fhl_award (Autodesk Fusion 360 design; units mm, degrees)
Autodesk Fusion 360 part; units mm, degrees
note: some values were not read from the file. Set by a fixed rule: which sketch regions a step uses.
(part 1 of 2)
sketch "Sketch1" plane through (0, 0, 0) normal (0, 1, 0) x (1, 0, 0)
  line L0 (0, 0) -> (-70, 0)
  line L1 (-70, 0) -> (-70, -200)
  line L2 (-70, -200) -> (0, -200)
  line L3 (0, -200) -> (0, 0)
  line L4 (-63, -200) -> (-7, -200)
  line L5 (-63, -200) -> (-11.8843, -162.1937)
  line L6 (-11.8843, -162.1937) -> (-35, -218)
  line L7 (-35, -218) -> (-66.1664, -152.3416)
  line L8 (-66.1664, -152.3416) -> (-7, -200)
  line L9 (-35, -218) -> (-35, -200)
  line L10 (-43.5442, -200) -> (-27.5442, -200)
  dimension "d1" = 70
  dimension "d2" = 200
  dimension "d3" = 7
  dimension "d4" = 7
  dimension "d5" = 18
  dimension "d6" = 16
  dimension "d7" = 112.5
  dimension "d9" = 101.095
  dimension "d10" = 106.351
  constraint horizontal L0
  constraint vertical L1
  constraint horizontal L2
  constraint vertical L3
  constraint coincident L0.start L3.end
  constraint coincident L2 L4.start
  constraint coincident L2 L4.end
  constraint perpendicular L2 L9
  constraint midpoint L2 L9.end
  constraint coincident L7 L10.start
  constraint coincident L6 L10.end
  constraint collinear L4 L10
  measures "d1" distance of L1.end L2.end
  measures "d2" distance of L0.start L2.end
  measures "d3" distance of L2.end L4.end
  measures "d4" distance of L1.end L4.start
  measures "d5" distance of L2 L6.end
  measures "d6" distance of L10.start L10.end
  measures "d7" angle of L2 L6
  measures "d9" angle of L5 L7
  measures "d10" angle of L6 L8
extrude "Extrude1" add sketch "Sketch1" along normal blind 48 contours L0 L1 L2 L3 L5 L6 L7 L8 | L2 L4 L6 L8 | L2 L4 L5 L7 | L2 L4 L5 L6 L7 L8 L10 | L5 L6 L8 | L5 L7 L8
extrude "Extrude2" add sketch "Sketch1" against normal blind 8 contours L2 L4 L6 L8 | L2 L4 L5 L7 | L2 L4 L6 L9 L10 | L2 L4 L5 L6 L7 L8 L10 | L5 L6 L8 | L2 L4 L7 L9 L10 | L5 L7 L8
sketch "Sketch2" plane through (-70, 0, 0) normal (-1, 0, 0) x (0, -1, 0)
  line L0 (0, 0) -> (0, 200)
  line L1 (0, 200) -> (-48, 200)
  line L2 (-48, 200) -> (-48, 0)
  line L3 (-48, 0) -> (0, 0)
  line L4 (-4, 200) -> (-48, 11.1856)
  line L5 (0, 0) -> (-48, 11.1856)
  line L6 (-4, 200) -> (-48, 200)
  line L7 (-48, 200) -> (-48, 0)
  line L8 (-48, 0) -> (0, 0)
  point P0 (0, 200)
  dimension "d15" = 90
  dimension "d16" = 4
  constraint coincident L1 L4.start
  constraint coincident L2 L4.end
  constraint coincident L0.start L3.end
  constraint coincident L1.end L2.start
  constraint coincident L2.end L3.start
  measures "d15" angle of L4 L5
  measures "d16" distance of L4.start P0
extrude "Extrude3" cut sketch "Sketch2" against normal blind 70 contours L2 L3 L5 L7 L8 | L1 L2 L4 L6 L7
fillet "Fillet1" radius 1 29 edges at (-70, 0, 100) (0, 26, 105.5928) (-35, 48, 11.1856) (-70, 26, 105.5928) (-70, 24, 5.5928) (-35, 4, 200) (-70, 2, 200) (0, 0, 100) (-3.5, 0, 200) (-7, -4, 200) (-63, -4, 200) (-66.5, 0, 200) (-55.7999, -8, 194.6746) (-53.2721, -8, 200) (-39.2721, -8, 209) (-35, -4, 218) (-39.2721, 0, 209) (-31.2721, 0, 209) (-31.2721, -8, 209) (-17.2721, -8, 200) (-14.7022, -8, 193.7959) (-57.3831, -8, 170.8455) (-49.9863, -8, 165.3746) (-22.8453, -8, 170.3007) (-17.1444, -8, 174.8927) (-66.1664, -4, 152.3416) (-11.8843, -4, 162.1937) (-35, 0, 0) (0, 24, 5.5928)
sketch "Sketch3" plane through (0, 0, 0) normal (0, -1, 0) x (1, 0, 0)
  line L0 (-1, 199) -> (-8.8356, 199)
  arc A0 (-9.2083, 198.2212) -> (-8.8356, 199) centre (-9.8356, 199) ccw
  line L1 (-9.2083, 198.2212) -> (-22.4045, 187.5917)
  line L2 (-22.4045, 187.5917) -> (-13.2636, 165.5237)
  arc A1 (-14.7821, 164.337) -> (-13.2636, 165.5237) centre (-14.1875, 165.141) ccw
  line L3 (-14.7821, 164.337) -> (-33.8062, 178.4077)
  line L4 (-33.8062, 178.4077) -> (-62.7601, 155.0854)
  arc A2 (-64.2908, 156.293) -> (-62.7601, 155.0854) centre (-63.3874, 155.8642) ccw
  line L5 (-64.2908, 156.293) -> (-48.5998, 189.3493)
  line L6 (-48.5998, 189.3493) -> (-60.5609, 198.196)
  arc A3 (-60.9663, 199) -> (-60.5609, 198.196) centre (-59.9663, 199) ccw
  line L7 (-60.9663, 199) -> (-69, 199)
  line L8 (-69, 199) -> (-69, 1.2598)
  line L9 (-69, 1.2598) -> (-1, 1.2598)
  line L10 (-1, 1.2598) -> (-1, 199)
  line L11 (-62.5, 91.2598) -> (-7.5, 91.2598)
  line L12 (-7.5, 91.2598) -> (-7.5, 71.2598)
  line L13 (-7.5, 71.2598) -> (-62.5, 71.2598)
  line L14 (-62.5, 71.2598) -> (-62.5, 91.2598)
  line L15 (-37.5, 101.2598) -> (-32.5, 101.2598)
  line L16 (-32.5, 101.2598) -> (-32.5, 61.2598)
  line L17 (-32.5, 61.2598) -> (-37.5, 61.2598)
  line L18 (-37.5, 61.2598) -> (-37.5, 101.2598)
  line L19 (-32.5, 61.2598) -> (-7.5, 71.2598)
  line L20 (-7.5, 91.2598) -> (-32.5, 101.2598)
  line L21 (-37.5, 101.2598) -> (-62.5, 91.2598)
  line L22 (-62.5, 71.2598) -> (-37.5, 61.2598)
  line L23 (-35, 101.2598) -> (-35, 61.2598)
  line L24 (-35, 61.2598) -> (-37.5, 61.2598)
  line L25 (-36.25, 61.2598) -> (-36.25, 71.2598)
  line L26 (-35, 61.2598) -> (-32.5, 61.2598)
  line L27 (-33.75, 61.2598) -> (-33.75, 71.2598)
  circle A4 centre (-35, 68.2598) radius 3
  line L28 (-35, 68.2598) -> (-36.25, 68.2598)
  line L29 (-35, 68.2598) -> (-33.75, 68.2598)
  line L30 (-50.0254, 86.3798) -> (-50.0254, 82.5627)
  line L31 (-50.0254, 82.5627) -> (-44.7683, 82.5627)
  line L32 (-44.7683, 82.5627) -> (-44.7683, 79.7284)
  line L33 (-44.7683, 79.7284) -> (-50.0254, 79.7284)
  line L34 (-50.0254, 79.7284) -> (-50.0254, 73.2598)
  line L35 (-50.0254, 73.2598) -> (-54.0254, 73.2598)
  line L36 (-54.0254, 73.2598) -> (-54.0254, 89.2598)
  line L37 (-54.0254, 89.2598) -> (-43.8083, 89.2598)
  line L38 (-43.8083, 89.2598) -> (-43.8083, 86.3798)
  line L39 (-43.8083, 86.3798) -> (-50.0254, 86.3798)
  line L40 (-28.5397, 73.2598) -> (-32.5397, 73.2598)
  line L41 (-32.5397, 73.2598) -> (-32.5397, 79.8884)
  line L42 (-32.5397, 79.8884) -> (-37.454, 79.8884)
  line L43 (-37.454, 79.8884) -> (-37.454, 73.2598)
  line L44 (-37.454, 73.2598) -> (-41.454, 73.2598)
  line L45 (-41.454, 73.2598) -> (-41.454, 89.2598)
  line L46 (-41.454, 89.2598) -> (-37.454, 89.2598)
  line L47 (-37.454, 89.2598) -> (-37.454, 82.9741)
  line L48 (-37.454, 82.9741) -> (-32.5397, 82.9741)
  line L49 (-32.5397, 82.9741) -> (-32.5397, 89.2598)
  line L50 (-32.5397, 89.2598) -> (-28.5397, 89.2598)
  line L51 (-28.5397, 89.2598) -> (-28.5397, 73.2598)
  line L52 (-14.5969, 76.2998) -> (-14.5969, 73.2598)
  line L53 (-14.5969, 73.2598) -> (-24.6083, 73.2598)
  line L54 (-24.6083, 73.2598) -> (-24.6083, 89.2598)
  line L55 (-24.6083, 89.2598) -> (-20.6083, 89.2598)
  line L56 (-20.6083, 89.2598) -> (-20.6083, 76.2998)
  line L57 (-20.6083, 76.2998) -> (-14.5969, 76.2998)
  dimension "d22" = 5
  dimension "d24" = 55
  dimension "d25" = 6.5
  dimension "d26" = 27.5
  dimension "d27" = 40
  dimension "d28" = 70
  dimension "d29" = 20
  dimension "d30" = 10
  dimension "d31" = 3
  constraint horizontal L11
  constraint vertical L12
  constraint horizontal L13
  constraint vertical L14
  constraint horizontal L15
  constraint vertical L16
  constraint horizontal L17
  constraint vertical L18
  constraint midpoint L15 L23.start
  constraint midpoint L17 L23.end
  constraint midpoint L24 L25.start
  constraint coincident L13 L25.end
  constraint perpendicular L13 L25
  constraint midpoint L26 L27.start
  constraint coincident L13 L27.end
  constraint perpendicular L13 L27
  constraint coincident L23 A4.centre
  constraint tangent L13 A4
  constraint coincident A4.centre L28.start
  constraint coincident L25 L28.end
  constraint perpendicular L25 L28
  constraint coincident L27 L29.end
  constraint perpendicular L27 L29
  measures "d22" distance of L16 L18
  measures "d24" distance of L12 L14
  measures "d25" distance of L10 L12
  measures "d26" distance of L12 L23
  measures "d27" distance of L23.start L23.end
  measures "d28" distance of L9 L13
  measures "d29" distance of L11.end L12.end
  measures "d30" distance of L13 L17
  measures "d31" distance of L13 A4.centre
extrude "Extrude4" cut sketch "Sketch3" against normal blind 2 contours L11 L18 L21 | L11 L13 L14 L18 L44 L45 L46 | L11 L15 L18 L23 | L11 L18 L23 L46 L47 L48 | L13 L18 L22 A4 | L11 L15 L16 L23 | L11 L16 L23 L48 L49 L50 | L13 L18 L23 L42 L43 L44 | L13 L18 L25 A4 | L17 L18 L24 L25 A4 | L11 L16 L20 | L11 L12 L13 L16 L40 L50 L51 | L13 L25 A4 | L13 L16 L23 L40 L41 L42 | L23 L27 A4 L29 | L13 L27 A4 | L23 L25 A4 L28 | L13 L16 L19 A4 | L13 L16 L27 A4 | L16 L17 L26 L27 A4 picked at (-34.1667, 69.1689) picked at (-35.8333, 69.1689)
fillet "Fillet3" radius 4 8 edges at (-62.5, 1, 71.2598) (-62.5, 1, 91.2598) (-37.5, 1, 101.2598) (-32.5, 1, 101.2598) (-7.5, 1, 91.2598) (-7.5, 1, 71.2598) (-32.5, 1, 61.2598) (-37.5, 1, 61.2598)
fillet "Fillet4" radius 0.7 4 edges at (-36.25, 1, 68.2598) (-33.75, 1, 68.2598) (-36.25, 1, 65.5326) (-33.75, 1, 65.5326)
fillet "Fillet5" radius 0.7 2 edges at (-33.75, 1, 61.2598) (-36.25, 1, 61.2598)
fillet "Fillet6" radius 0.1 2 edges at (-36.25, 1, 70.987) (-33.75, 1, 70.987)
fillet "Fillet7" radius 0.25 28 edges at (-28.5397, 1, 73.2598) (-32.5397, 1, 73.2598) (-37.454, 1, 73.2598) (-37.454, 1, 79.8884) (-32.5397, 1, 79.8884) (-41.454, 1, 73.2598) (-41.454, 1, 89.2598) (-37.454, 1, 89.2598) (-37.454, 1, 82.9741) (-32.5397, 1, 82.9741) (-32.5397, 1, 89.2598) (-28.5397, 1, 89.2598) (-24.6083, 1, 89.2598) (-20.6083, 1, 89.2598) (-20.6083, 1, 76.2998) (-14.5969, 1, 76.2998) (-14.5969, 1, 73.2598) (-24.6083, 1, 73.2598) (-54.0254, 1, 73.2598) (-54.0254, 1, 89.2598) (-43.8083, 1, 89.2598) (-43.8083, 1, 86.3798) (-50.0254, 1, 82.5627) (-44.7683, 1, 82.5627) (-50.0254, 1, 86.3798) (-44.7683, 1, 79.7284) (-50.0254, 1, 79.7284) (-50.0254, 1, 73.2598)
sketch "Sketch4" plane through (0, 0, 0) normal (0, -1, 0) x (1, 0, 0)
  line L0 (-1, 199) -> (-8.8356, 199)
  arc A0 (-9.2083, 198.2212) -> (-8.8356, 199) centre (-9.8356, 199) ccw
  line L1 (-9.2083, 198.2212) -> (-22.4045, 187.5917)
  line L2 (-22.4045, 187.5917) -> (-13.2636, 165.5237)
  arc A1 (-14.7821, 164.337) -> (-13.2636, 165.5237) centre (-14.1875, 165.141) ccw
  line L3 (-14.7821, 164.337) -> (-33.8062, 178.4077)
  line L4 (-33.8062, 178.4077) -> (-62.7601, 155.0854)
  arc A2 (-64.2908, 156.293) -> (-62.7601, 155.0854) centre (-63.3874, 155.8642) ccw
  line L5 (-64.2908, 156.293) -> (-48.5998, 189.3493)
  line L6 (-48.5998, 189.3493) -> (-60.5609, 198.196)
  arc A3 (-60.9663, 199) -> (-60.5609, 198.196) centre (-59.9663, 199) ccw
  line L7 (-60.9663, 199) -> (-69, 199)
  line L8 (-69, 199) -> (-69, 1.2598)
  line L9 (-69, 1.2598) -> (-1, 1.2598)
  line L10 (-1, 1.2598) -> (-1, 199)
  arc A4 (-33.6034, 70.9149) -> (-33.75, 70.8264) centre (-33.65, 70.8264) ccw
  line L11 (-33.75, 70.8264) -> (-33.75, 68.9598)
  arc A5 (-34.45, 68.2598) -> (-33.75, 68.9598) centre (-34.45, 68.9598) ccw
  line L12 (-34.45, 68.2598) -> (-35.55, 68.2598)
  arc A6 (-36.25, 68.9598) -> (-35.55, 68.2598) centre (-35.55, 68.9598) ccw
  line L13 (-36.25, 68.9598) -> (-36.25, 70.8264)
  arc A7 (-36.25, 70.8264) -> (-36.3966, 70.9149) centre (-36.35, 70.8264) ccw
  arc A8 (-36.3966, 70.9149) -> (-36.5811, 65.7103) centre (-35, 68.2598) ccw
  arc A9 (-36.25, 65.1154) -> (-36.5811, 65.7103) centre (-36.95, 65.1154) ccw
  line L14 (-36.25, 65.1154) -> (-36.25, 61.9672)
  arc A10 (-36.9967, 61.2688) -> (-36.25, 61.9672) centre (-36.95, 61.9672) ccw
  arc A11 (-38.2152, 61.5459) -> (-36.9967, 61.2688) centre (-36.7297, 65.2598) ccw
  line L15 (-38.2152, 61.5459) -> (-59.9856, 70.2541)
  arc A12 (-62.5, 73.968) -> (-59.9856, 70.2541) centre (-58.5, 73.968) ccw
  line L16 (-62.5, 73.968) -> (-62.5, 88.5517)
  arc A13 (-59.9856, 92.2656) -> (-62.5, 88.5517) centre (-58.5, 88.5517) ccw
  line L17 (-59.9856, 92.2656) -> (-38.2152, 100.9737)
  arc A14 (-36.7297, 101.2598) -> (-38.2152, 100.9737) centre (-36.7297, 97.2598) ccw
  line L18 (-36.7297, 101.2598) -> (-33.2703, 101.2598)
  arc A15 (-31.7848, 100.9737) -> (-33.2703, 101.2598) centre (-33.2703, 97.2598) ccw
  line L19 (-31.7848, 100.9737) -> (-10.0144, 92.2656)
  arc A16 (-7.5, 88.5517) -> (-10.0144, 92.2656) centre (-11.5, 88.5517) ccw
  line L20 (-7.5, 88.5517) -> (-7.5, 73.968)
  arc A17 (-10.0144, 70.2541) -> (-7.5, 73.968) centre (-11.5, 73.968) ccw
  line L21 (-10.0144, 70.2541) -> (-31.7848, 61.5459)
  arc A18 (-33.0033, 61.2688) -> (-31.7848, 61.5459) centre (-33.2703, 65.2598) ccw
  arc A19 (-33.75, 61.9672) -> (-33.0033, 61.2688) centre (-33.05, 61.9672) ccw
  line L22 (-33.75, 61.9672) -> (-33.75, 65.1154)
  arc A20 (-33.4189, 65.7103) -> (-33.75, 65.1154) centre (-33.05, 65.1154) ccw
  arc A21 (-33.4189, 65.7103) -> (-33.6034, 70.9149) centre (-35, 68.2598) ccw
  line L23 (-69, 1.2598) -> (-1, 1.2598)
  line L24 (-1, 1.2598) -> (-1, 61.2598)
  line L25 (-1, 61.2598) -> (-69, 61.2598)
  line L26 (-69, 61.2598) -> (-69, 1.2598)
  line L27 (-35, 1.2598) -> (-35, 61.2598)
  line L28 (-41.8, 61.2598) -> (-41.8, 1.2598)
  line L29 (-48.6, 1.2598) -> (-48.6, 61.2598)
  line L30 (-55.4, 61.2598) -> (-55.4, 1.2598)
  line L31 (-62.2, 1.2598) -> (-62.2, 61.2598)
  line L32 (-28.2, 61.2598) -> (-28.2, 1.2598)
  line L33 (-21.4, 1.2598) -> (-21.4, 61.2598)
  line L34 (-14.6, 61.2598) -> (-14.6, 1.2598)
  line L35 (-7.8, 1.2598) -> (-7.8, 61.2598)
  line L36 (-58.2383, 47.7567) -> (-55.6853, 47.7567)
  spline S0 degree 2 poles (-55.6853, 47.7567) (-55.1681, 47.7567) (-54.8848, 48.007) knots 0 0 0 1 1 1
  spline S1 degree 2 poles (-54.8848, 48.007) (-54.6014, 48.2574) (-54.6014, 48.7086) knots 0 0 0 1 1 1
  line L37 (-54.6014, 48.7086) -> (-54.6014, 48.7251)
  spline S2 degree 2 poles (-54.6014, 48.7251) (-54.6014, 49.0277) (-54.728, 49.2423) knots 0 0 0 1 1 1
  spline S3 degree 2 poles (-54.728, 49.2423) (-54.8545, 49.4568) (-55.0993, 49.5696) knots 0 0 0 1 1 1
  spline S4 degree 2 poles (-55.0993, 49.5696) (-55.3442, 49.6824) (-55.6853, 49.6824) knots 0 0 0 1 1 1
  line L38 (-55.6853, 49.6824) -> (-58.2383, 49.6824)
  line L39 (-58.2383, 49.6824) -> (-58.2383, 51.135)
  line L40 (-58.2383, 51.135) -> (-55.6853, 51.135)
  spline S5 degree 2 poles (-55.6853, 51.135) (-55.2176, 51.135) (-54.9618, 51.3716) knots 0 0 0 1 1 1
  spline S6 degree 2 poles (-54.9618, 51.3716) (-54.706, 51.6081) (-54.706, 52.0373) knots 0 0 0 1 1 1
  spline S7 degree 2 poles (-54.706, 52.0373) (-54.706, 52.4224) (-54.9618, 52.637) knots 0 0 0 1 1 1
  spline S8 degree 2 poles (-54.9618, 52.637) (-55.2176, 52.8516) (-55.6853, 52.8516) knots 0 0 0 1 1 1
  line L41 (-55.6853, 52.8516) -> (-58.2383, 52.8516)
  line L42 (-58.2383, 52.8516) -> (-58.2383, 54.3042)
  line L43 (-58.2383, 54.3042) -> (-55.6358, 54.3042)
  spline S9 degree 2 poles (-55.6358, 54.3042) (-54.86, 54.3042) (-54.3098, 54.0483) knots 0 0 0 1 1 1
  spline S10 degree 2 poles (-54.3098, 54.0483) (-53.7596, 53.7925) (-53.4735, 53.3055) knots 0 0 0 1 1 1
  spline S11 degree 2 poles (-53.4735, 53.3055) (-53.1874, 52.8186) (-53.1874, 52.1363) knots 0 0 0 1 1 1
  spline S12 degree 2 poles (-53.1874, 52.1363) (-53.1874, 51.6687) (-53.3717, 51.3083) knots 0 0 0 1 1 1
  spline S13 degree 2 poles (-53.3717, 51.3083) (-53.556, 50.9479) (-53.9082, 50.7168) knots 0 0 0 1 1 1
  spline S14 degree 2 poles (-53.9082, 50.7168) (-54.2603, 50.4857) (-54.7555, 50.4032) knots 0 0 0 1 1 1
  spline S15 degree 2 poles (-54.7555, 50.4032) (-54.2273, 50.3317) (-53.8504, 50.0813) knots 0 0 0 1 1 1
  spline S16 degree 2 poles (-53.8504, 50.0813) (-53.4735, 49.831) (-53.2782, 49.4293) knots 0 0 0 1 1 1
  spline S17 degree 2 poles (-53.2782, 49.4293) (-53.0828, 49.0277) (-53.0828, 48.4995) knots 0 0 0 1 1 1
  line L44 (-53.0828, 48.4995) -> (-53.0828, 48.483)
  spline S18 degree 2 poles (-53.0828, 48.483) (-53.0828, 47.7952) (-53.3717, 47.3055) knots 0 0 0 1 1 1
  spline S19 degree 2 poles (-53.3717, 47.3055) (-53.6606, 46.8158) (-54.2135, 46.56) knots 0 0 0 1 1 1
  spline S20 degree 2 poles (-54.2135, 46.56) (-54.7665, 46.3042) (-55.5423, 46.3042) knots 0 0 0 1 1 1
  line L45 (-55.5423, 46.3042) -> (-58.2383, 46.3042)
  line L46 (-58.2383, 46.3042) -> (-58.2383, 47.7567)
  line L47 (-58.8985, 54.3042) -> (-57.391, 54.3042)
  line L48 (-57.391, 54.3042) -> (-57.391, 46.3042)
  line L49 (-57.391, 46.3042) -> (-58.8985, 46.3042)
  line L50 (-58.8985, 46.3042) -> (-58.8985, 54.3042)
  spline S21 degree 2 poles (-49.2864, 46.2216) (-50.1117, 46.2216) (-50.6977, 46.5215) knots 0 0 0 1 1 1
  spline S22 degree 2 poles (-50.6977, 46.5215) (-51.2837, 46.8213) (-51.5918, 47.3963) knots 0 0 0 1 1 1
  spline S23 degree 2 poles (-51.5918, 47.3963) (-51.8999, 47.9713) (-51.8999, 48.7801) knots 0 0 0 1 1 1
  line L51 (-51.8999, 48.7801) -> (-51.8999, 49.4238)
  spline S24 degree 2 poles (-51.8999, 49.4238) (-51.8999, 50.2711) (-51.6055, 50.8709) knots 0 0 0 1 1 1
  spline S25 degree 2 poles (-51.6055, 50.8709) (-51.3112, 51.4706) (-50.7472, 51.7842) knots 0 0 0 1 1 1
  spline S26 degree 2 poles (-50.7472, 51.7842) (-50.1833, 52.0978) (-49.3855, 52.0978) knots 0 0 0 1 1 1
  spline S27 degree 2 poles (-49.3855, 52.0978) (-48.6372, 52.0978) (-48.1035, 51.7237) knots 0 0 0 1 1 1
  spline S28 degree 2 poles (-48.1035, 51.7237) (-47.5698, 51.3495) (-47.2919, 50.637) knots 0 0 0 1 1 1
  spline S29 degree 2 poles (-47.2919, 50.637) (-47.0141, 49.9245) (-47.0141, 48.9176) knots 0 0 0 1 1 1
  line L52 (-47.0141, 48.9176) -> (-47.0141, 48.5435)
  line L53 (-47.0141, 48.5435) -> (-50.9205, 48.5435)
  line L54 (-50.9205, 48.5435) -> (-50.9205, 49.5614)
  line L55 (-50.9205, 49.5614) -> (-48.3896, 49.5614)
  line L56 (-48.3896, 49.5614) -> (-48.4061, 49.6934)
  spline S30 degree 2 poles (-48.4061, 49.6934) (-48.4666, 50.1886) (-48.717, 50.4582) knots 0 0 0 1 1 1
  spline S31 degree 2 poles (-48.717, 50.4582) (-48.9673, 50.7278) (-49.3855, 50.7278) knots 0 0 0 1 1 1
  spline S32 degree 2 poles (-49.3855, 50.7278) (-49.9302, 50.7278) (-50.23, 50.4032) knots 0 0 0 1 1 1
  spline S33 degree 2 poles (-50.23, 50.4032) (-50.5299, 50.0786) (-50.5299, 49.4843) knots 0 0 0 1 1 1
  line L57 (-50.5299, 49.4843) -> (-50.5299, 48.7581)
  spline S34 degree 2 poles (-50.5299, 48.7581) (-50.5299, 48.1749) (-50.2025, 47.8557) knots 0 0 0 1 1 1
  spline S35 degree 2 poles (-50.2025, 47.8557) (-49.8751, 47.5366) (-49.2864, 47.5366) knots 0 0 0 1 1 1
  spline S36 degree 2 poles (-49.2864, 47.5366) (-48.9838, 47.5366) (-48.6867, 47.6439) knots 0 0 0 1 1 1
  spline S37 degree 2 poles (-48.6867, 47.6439) (-48.3896, 47.7512) (-48.1475, 47.9493) knots 0 0 0 1 1 1
  line L58 (-48.1475, 47.9493) -> (-47.1626, 47.0744)
  spline S38 degree 2 poles (-47.1626, 47.0744) (-47.6083, 46.6673) (-48.164, 46.4445) knots 0 0 0 1 1 1
  spline S39 degree 2 poles (-48.164, 46.4445) (-48.7197, 46.2216) (-49.2864, 46.2216) knots 0 0 0 1 1 1
  spline S40 degree 2 poles (-43.5093, 46.2216) (-44.0209, 46.2216) (-44.5051, 46.3124) knots 0 0 0 1 1 1
  spline S41 degree 2 poles (-44.5051, 46.3124) (-44.9893, 46.4032) (-45.413, 46.5793) knots 0 0 0 1 1 1
  spline S42 degree 2 poles (-45.413, 46.5793) (-45.8366, 46.7553) (-46.1612, 47.0029) knots 0 0 0 1 1 1
  line L59 (-46.1612, 47.0029) -> (-45.2314, 48.1639)
  spline S43 degree 2 poles (-45.2314, 48.1639) (-44.8187, 47.8998) (-44.3676, 47.7567) knots 0 0 0 1 1 1
  spline S44 degree 2 poles (-44.3676, 47.7567) (-43.9164, 47.6136) (-43.5093, 47.6136) knots 0 0 0 1 1 1
  spline S45 degree 2 poles (-43.5093, 47.6136) (-42.9811, 47.6136) (-42.6894, 47.7319) knots 0 0 0 1 1 1
  spline S46 degree 2 poles (-42.6894, 47.7319) (-42.3978, 47.8502) (-42.3978, 48.0593) knots 0 0 0 1 1 1
  spline S47 degree 2 poles (-42.3978, 48.0593) (-42.3978, 48.2519) (-42.5244, 48.3509) knots 0 0 0 1 1 1
  spline S48 degree 2 poles (-42.5244, 48.3509) (-42.6509, 48.45) (-42.849, 48.4912) knots 0 0 0 1 1 1
  spline S49 degree 2 poles (-42.849, 48.4912) (-43.0471, 48.5325) (-43.4047, 48.5655) knots 0 0 0 1 1 1
  spline S50 degree 2 poles (-43.4047, 48.5655) (-43.5037, 48.5765) (-43.6055, 48.5875) knots 0 0 0 1 1 1
  spline S51 degree 2 poles (-43.6055, 48.5875) (-43.7073, 48.5985) (-43.8119, 48.6095) knots 0 0 0 1 1 1
  spline S52 degree 2 poles (-43.8119, 48.6095) (-43.8339, 48.615) (-43.8586, 48.6178) knots 0 0 0 1 1 1
  spline S53 degree 2 poles (-43.8586, 48.6178) (-43.8834, 48.6205) (-43.9054, 48.6205) knots 0 0 0 1 1 1
  spline S54 degree 2 poles (-43.9054, 48.6205) (-44.5436, 48.7031) (-44.9288, 48.8241) knots 0 0 0 1 1 1
  spline S55 degree 2 poles (-44.9288, 48.8241) (-45.3139, 48.9451) (-45.5808, 49.289) knots 0 0 0 1 1 1
  spline S56 degree 2 poles (-45.5808, 49.289) (-45.8476, 49.6329) (-45.8476, 50.2876) knots 0 0 0 1 1 1
  spline S57 degree 2 poles (-45.8476, 50.2876) (-45.8476, 50.8599) (-45.5725, 51.267) knots 0 0 0 1 1 1
  spline S58 degree 2 poles (-45.5725, 51.267) (-45.2974, 51.6742) (-44.7747, 51.886) knots 0 0 0 1 1 1
  spline S59 degree 2 poles (-44.7747, 51.886) (-44.252, 52.0978) (-43.5093, 52.0978) knots 0 0 0 1 1 1
  spline S60 degree 2 poles (-43.5093, 52.0978) (-43.0746, 52.0978) (-42.6427, 52.0098) knots 0 0 0 1 1 1
  spline S61 degree 2 poles (-42.6427, 52.0098) (-42.2108, 51.9218) (-41.8146, 51.7567) knots 0 0 0 1 1 1
  spline S62 degree 2 poles (-41.8146, 51.7567) (-41.4185, 51.5916) (-41.0828, 51.3606) knots 0 0 0 1 1 1
  line L60 (-41.0828, 51.3606) -> (-41.9797, 50.2656)
  spline S63 degree 2 poles (-41.9797, 50.2656) (-42.3538, 50.4747) (-42.761, 50.5903) knots 0 0 0 1 1 1
  spline S64 degree 2 poles (-42.761, 50.5903) (-43.1681, 50.7058) (-43.5423, 50.7058) knots 0 0 0 1 1 1
  spline S65 degree 2 poles (-43.5423, 50.7058) (-43.9989, 50.7058) (-44.252, 50.6013) knots 0 0 0 1 1 1
  spline S66 degree 2 poles (-44.252, 50.6013) (-44.5051, 50.4967) (-44.5051, 50.3097) knots 0 0 0 1 1 1
  spline S67 degree 2 poles (-44.5051, 50.3097) (-44.5051, 50.1666) (-44.3703, 50.0868) knots 0 0 0 1 1 1
  spline S68 degree 2 poles (-44.3703, 50.0868) (-44.2355, 50.007) (-44.0347, 49.9713) knots 0 0 0 1 1 1
  spline S69 degree 2 poles (-44.0347, 49.9713) (-43.8339, 49.9355) (-43.4487, 49.8915) knots 0 0 0 1 1 1
  spline S70 degree 2 poles (-43.4487, 49.8915) (-43.3992, 49.886) (-43.3497, 49.8805) knots 0 0 0 1 1 1
  spline S71 degree 2 poles (-43.3497, 49.8805) (-43.3002, 49.875) (-43.2507, 49.8695) knots 0 0 0 1 1 1
  spline S72 degree 2 poles (-43.2507, 49.8695) (-43.2286, 49.864) (-43.2011, 49.864) knots 0 0 0 1 1 1
  spline S73 degree 2 poles (-43.2011, 49.864) (-43.1736, 49.864) (-43.1516, 49.8585) knots 0 0 0 1 1 1
  spline S74 degree 2 poles (-43.1516, 49.8585) (-42.4859, 49.7815) (-42.0677, 49.6604) knots 0 0 0 1 1 1
  spline S75 degree 2 poles (-42.0677, 49.6604) (-41.6496, 49.5394) (-41.3552, 49.1762) knots 0 0 0 1 1 1
  spline S76 degree 2 poles (-41.3552, 49.1762) (-41.0608, 48.8131) (-41.0608, 48.1088) knots 0 0 0 1 1 1
  spline S77 degree 2 poles (-41.0608, 48.1088) (-41.0608, 47.5146) (-41.3469, 47.0909) knots 0 0 0 1 1 1
  spline S78 degree 2 poles (-41.3469, 47.0909) (-41.6331, 46.6673) (-42.1833, 46.4445) knots 0 0 0 1 1 1
  spline S79 degree 2 poles (-42.1833, 46.4445) (-42.7335, 46.2216) (-43.5093, 46.2216) knots 0 0 0 1 1 1
  spline S80 degree 2 poles (-38.2548, 46.2766) (-39.0031, 46.2766) (-39.3524, 46.659) knots 0 0 0 1 1 1
  spline S81 degree 2 poles (-39.3524, 46.659) (-39.7018, 47.0414) (-39.7018, 47.7897) knots 0 0 0 1 1 1
  line L61 (-39.7018, 47.7897) -> (-39.7018, 53.6769)
  line L62 (-39.7018, 53.6769) -> (-38.1943, 53.6769)
  line L63 (-38.1943, 53.6769) -> (-38.1943, 48.1639)
  spline S82 degree 2 poles (-38.1943, 48.1639) (-38.1943, 47.9548) (-38.1117, 47.842) knots 0 0 0 1 1 1
  spline S83 degree 2 poles (-38.1117, 47.842) (-38.0292, 47.7292) (-37.8696, 47.7292) knots 0 0 0 1 1 1
  line L64 (-37.8696, 47.7292) -> (-37.4955, 47.7292)
  line L65 (-37.4955, 47.7292) -> (-37.4955, 46.2766)
  line L66 (-37.4955, 46.2766) -> (-38.2548, 46.2766)
  line L67 (-40.2905, 52.0153) -> (-37.4955, 52.0153)
  line L68 (-37.4955, 52.0153) -> (-37.4955, 50.7278)
  line L69 (-37.4955, 50.7278) -> (-40.2905, 50.7278)
  line L70 (-40.2905, 50.7278) -> (-40.2905, 52.0153)
  line L71 (-28.6592, 54.3042) -> (-27.1516, 54.3042)
  line L72 (-27.1516, 54.3042) -> (-27.1516, 46.3042)
  line L73 (-27.1516, 46.3042) -> (-28.6592, 46.3042)
  line L74 (-28.6592, 46.3042) -> (-28.6592, 54.3042)
  line L75 (-33.0388, 54.3042) -> (-31.5313, 54.3042)
  line L76 (-31.5313, 54.3042) -> (-31.5313, 46.3042)
  line L77 (-31.5313, 46.3042) -> (-33.0388, 46.3042)
  line L78 (-33.0388, 46.3042) -> (-33.0388, 54.3042)
  line L79 (-32.3401, 50.9974) -> (-27.6798, 50.9974)
  line L80 (-27.6798, 50.9974) -> (-27.6798, 49.5449)
  line L81 (-27.6798, 49.5449) -> (-32.3401, 49.5449)
  line L82 (-32.3401, 49.5449) -> (-32.3401, 50.9974)
  spline S84 degree 2 poles (-22.3593, 49.9245) (-22.3593, 50.3207) (-22.6234, 50.5352) knots 0 0 0 1 1 1
  spline S85 degree 2 poles (-22.6234, 50.5352) (-22.8875, 50.7498) (-23.3717, 50.7498) knots 0 0 0 1 1 1
  spline S86 degree 2 poles (-23.3717, 50.7498) (-23.6908, 50.7498) (-24.0044, 50.6453) knots 0 0 0 1 1 1
  spline S87 degree 2 poles (-24.0044, 50.6453) (-24.3181, 50.5407) (-24.5601, 50.3537) knots 0 0 0 1 1 1
  line L83 (-24.5601, 50.3537) -> (-25.4955, 51.2725)
  spline S88 degree 2 poles (-25.4955, 51.2725) (-25.1544, 51.6632) (-24.5932, 51.8805) knots 0 0 0 1 1 1
  spline S89 degree 2 poles (-24.5932, 51.8805) (-24.032, 52.0978) (-23.3497, 52.0978) knots 0 0 0 1 1 1
  spline S90 degree 2 poles (-23.3497, 52.0978) (-22.6014, 52.0978) (-22.0732, 51.8475) knots 0 0 0 1 1 1
  spline S91 degree 2 poles (-22.0732, 51.8475) (-21.545, 51.5971) (-21.2672, 51.1212) knots 0 0 0 1 1 1
  spline S92 degree 2 poles (-21.2672, 51.1212) (-20.9893, 50.6453) (-20.9893, 49.974) knots 0 0 0 1 1 1
  line L84 (-20.9893, 49.974) -> (-20.9893, 46.3042)
  line L85 (-20.9893, 46.3042) -> (-22.3593, 46.3042)
  line L86 (-22.3593, 46.3042) -> (-22.3593, 49.9245)
  spline S93 degree 2 poles (-23.9494, 46.2216) (-24.8683, 46.2216) (-25.3222, 46.659) knots 0 0 0 1 1 1
  spline S94 degree 2 poles (-25.3222, 46.659) (-25.7761, 47.0965) (-25.7761, 47.9878) knots 0 0 0 1 1 1
  spline S95 degree 2 poles (-25.7761, 47.9878) (-25.7761, 48.8351) (-25.2672, 49.2588) knots 0 0 0 1 1 1
  spline S96 degree 2 poles (-25.2672, 49.2588) (-24.7582, 49.6824) (-23.7403, 49.6824) knots 0 0 0 1 1 1
  line L87 (-23.7403, 49.6824) -> (-22.3098, 49.6824)
  line L88 (-22.3098, 49.6824) -> (-22.2328, 48.5325)
  line L89 (-22.2328, 48.5325) -> (-23.7348, 48.5325)
  spline S97 degree 2 poles (-23.7348, 48.5325) (-24.076, 48.5325) (-24.2465, 48.3977) knots 0 0 0 1 1 1
  spline S98 degree 2 poles (-24.2465, 48.3977) (-24.4171, 48.2629) (-24.4171, 47.9878) knots 0 0 0 1 1 1
  spline S99 degree 2 poles (-24.4171, 47.9878) (-24.4171, 47.7072) (-24.2025, 47.5724) knots 0 0 0 1 1 1
  spline S100 degree 2 poles (-24.2025, 47.5724) (-23.9879, 47.4376) (-23.5533, 47.4376) knots 0 0 0 1 1 1
  spline S101 degree 2 poles (-23.5533, 47.4376) (-22.948, 47.4376) (-22.6537, 47.5751) knots 0 0 0 1 1 1
  spline S102 degree 2 poles (-22.6537, 47.5751) (-22.3593, 47.7127) (-22.3593, 48.0043) knots 0 0 0 1 1 1
  line L90 (-22.3593, 48.0043) -> (-22.2438, 47.1735)
  spline S103 degree 2 poles (-22.2438, 47.1735) (-22.2768, 46.8654) (-22.5271, 46.6508) knots 0 0 0 1 1 1
  spline S104 degree 2 poles (-22.5271, 46.6508) (-22.7775, 46.4362) (-23.1544, 46.3289) knots 0 0 0 1 1 1
  spline S105 degree 2 poles (-23.1544, 46.3289) (-23.5313, 46.2216) (-23.9494, 46.2216) knots 0 0 0 1 1 1
  spline S106 degree 2 poles (-17.0883, 46.2216) (-17.9026, 46.2216) (-18.4831, 46.5325) knots 0 0 0 1 1 1
  spline S107 degree 2 poles (-18.4831, 46.5325) (-19.0636, 46.8434) (-19.3662, 47.4376) knots 0 0 0 1 1 1
  spline S108 degree 2 poles (-19.3662, 47.4376) (-19.6688, 48.0318) (-19.6688, 48.8681) knots 0 0 0 1 1 1
  line L91 (-19.6688, 48.8681) -> (-19.6688, 49.4788)
  spline S109 degree 2 poles (-19.6688, 49.4788) (-19.6688, 50.3097) (-19.3662, 50.8956) knots 0 0 0 1 1 1
  spline S110 degree 2 poles (-19.3662, 50.8956) (-19.0636, 51.4816) (-18.4831, 51.7897) knots 0 0 0 1 1 1
  spline S111 degree 2 poles (-18.4831, 51.7897) (-17.9026, 52.0978) (-17.0883, 52.0978) knots 0 0 0 1 1 1
  spline S112 degree 2 poles (-17.0883, 52.0978) (-16.6207, 52.0978) (-16.2053, 51.9905) knots 0 0 0 1 1 1
  spline S113 degree 2 poles (-16.2053, 51.9905) (-15.7899, 51.8832) (-15.4597, 51.6797) knots 0 0 0 1 1 1
  spline S114 degree 2 poles (-15.4597, 51.6797) (-15.1296, 51.4761) (-14.9095, 51.1845) knots 0 0 0 1 1 1
  line L92 (-14.9095, 51.1845) -> (-15.8834, 50.2381)
  spline S115 degree 2 poles (-15.8834, 50.2381) (-16.0925, 50.4307) (-16.3731, 50.538) knots 0 0 0 1 1 1
  spline S116 degree 2 poles (-16.3731, 50.538) (-16.6537, 50.6453) (-16.9618, 50.6453) knots 0 0 0 1 1 1
  spline S117 degree 2 poles (-16.9618, 50.6453) (-17.534, 50.6453) (-17.8476, 50.3399) knots 0 0 0 1 1 1
  spline S118 degree 2 poles (-17.8476, 50.3399) (-18.1612, 50.0346) (-18.1612, 49.4788) knots 0 0 0 1 1 1
  line L93 (-18.1612, 49.4788) -> (-18.1612, 48.8681)
  spline S119 degree 2 poles (-18.1612, 48.8681) (-18.1612, 48.2959) (-17.8476, 47.985) knots 0 0 0 1 1 1
  spline S120 degree 2 poles (-17.8476, 47.985) (-17.534, 47.6742) (-16.9618, 47.6742) knots 0 0 0 1 1 1
  spline S121 degree 2 poles (-16.9618, 47.6742) (-16.6482, 47.6742) (-16.3676, 47.7897) knots 0 0 0 1 1 1
  spline S122 degree 2 poles (-16.3676, 47.7897) (-16.087, 47.9053) (-15.8834, 48.1198) knots 0 0 0 1 1 1
  line L94 (-15.8834, 48.1198) -> (-14.9095, 47.1185)
  spline S123 degree 2 poles (-14.9095, 47.1185) (-15.1351, 46.8324) (-15.4652, 46.6315) knots 0 0 0 1 1 1
  spline S124 degree 2 poles (-15.4652, 46.6315) (-15.7954, 46.4307) (-16.208, 46.3262) knots 0 0 0 1 1 1
  spline S125 degree 2 poles (-16.208, 46.3262) (-16.6207, 46.2216) (-17.0883, 46.2216) knots 0 0 0 1 1 1
  line L95 (-13.1874, 48.3619) -> (-10.5244, 52.0153)
  line L96 (-10.5244, 52.0153) -> (-8.9288, 52.0153)
  line L97 (-8.9288, 52.0153) -> (-12.9838, 46.7003)
  line L98 (-12.9838, 46.7003) -> (-13.1874, 48.3619)
  line L99 (-13.8916, 54.3042) -> (-12.3841, 54.3042)
  line L100 (-12.3841, 54.3042) -> (-12.3841, 46.3042)
  line L101 (-12.3841, 46.3042) -> (-13.8916, 46.3042)
  line L102 (-13.8916, 46.3042) -> (-13.8916, 54.3042)
  line L103 (-11.8339, 49.2533) -> (-10.5904, 50.0015)
  line L104 (-10.5904, 50.0015) -> (-8.6482, 46.3042)
  line L105 (-8.6482, 46.3042) -> (-10.3923, 46.3042)
  line L106 (-10.3923, 46.3042) -> (-11.8339, 49.2533)
  line L107 (-45.7023, 36.4913) -> (-43.1284, 39.875)
  spline S126 degree 2 poles (-43.1284, 39.875) (-42.953, 40.102) (-42.8576, 40.3418) knots 0 0 0 1 1 1
  spline S127 degree 2 poles (-42.8576, 40.3418) (-42.7622, 40.5817) (-42.7622, 40.788) knots 0 0 0 1 1 1
  line L108 (-42.7622, 40.788) -> (-42.7622, 40.7983)
  spline S128 degree 2 poles (-42.7622, 40.7983) (-42.7622, 41.1027) (-42.9582, 41.2677) knots 0 0 0 1 1 1
  spline S129 degree 2 poles (-42.9582, 41.2677) (-43.1542, 41.4328) (-43.5153, 41.4328) knots 0 0 0 1 1 1
  spline S130 degree 2 poles (-43.5153, 41.4328) (-43.866, 41.4328) (-44.0827, 41.2033) knots 0 0 0 1 1 1
  spline S131 degree 2 poles (-44.0827, 41.2033) (-44.2993, 40.9737) (-44.3457, 40.5508) knots 0 0 0 1 1 1
  line L109 (-44.3457, 40.5508) -> (-44.3457, 40.5456)
  line L110 (-44.3457, 40.5456) -> (-45.7952, 40.5456)
  line L111 (-45.7952, 40.5456) -> (-45.7952, 40.5508)
  spline S132 degree 2 poles (-45.7952, 40.5508) (-45.7488, 41.2523) (-45.4573, 41.7578) knots 0 0 0 1 1 1
  spline S133 degree 2 poles (-45.4573, 41.7578) (-45.1659, 42.2633) (-44.6707, 42.5289) knots 0 0 0 1 1 1
  spline S134 degree 2 poles (-44.6707, 42.5289) (-44.1755, 42.7946) (-43.5256, 42.7946) knots 0 0 0 1 1 1
  spline S135 degree 2 poles (-43.5256, 42.7946) (-42.8241, 42.7946) (-42.3263, 42.565) knots 0 0 0 1 1 1
  spline S136 degree 2 poles (-42.3263, 42.565) (-41.8285, 42.3355) (-41.5681, 41.897) knots 0 0 0 1 1 1
  spline S137 degree 2 poles (-41.5681, 41.897) (-41.3076, 41.4586) (-41.3076, 40.8396) knots 0 0 0 1 1 1
  line L112 (-41.3076, 40.8396) -> (-41.3076, 40.8345)
  spline S138 degree 2 poles (-41.3076, 40.8345) (-41.3076, 40.3238) (-41.4855, 39.8209) knots 0 0 0 1 1 1
  spline S139 degree 2 poles (-41.4855, 39.8209) (-41.6635, 39.3179) (-41.9833, 38.9105) knots 0 0 0 1 1 1
  line L113 (-41.9833, 38.9105) -> (-43.8299, 36.579)
  line L114 (-43.8299, 36.579) -> (-41.2663, 36.579)
  line L115 (-41.2663, 36.579) -> (-41.2663, 35.2172)
  line L116 (-41.2663, 35.2172) -> (-45.7023, 35.2172)
  line L117 (-45.7023, 35.2172) -> (-45.7023, 36.4913)
  spline S140 degree 2 poles (-37.8877, 35.1398) (-38.9864, 35.1398) (-39.5589, 35.7046) knots 0 0 0 1 1 1
  spline S141 degree 2 poles (-39.5589, 35.7046) (-40.1315, 36.2695) (-40.1315, 37.2701) knots 0 0 0 1 1 1
  line L118 (-40.1315, 37.2701) -> (-40.1315, 40.6797)
  spline S142 degree 2 poles (-40.1315, 40.6797) (-40.1315, 41.6907) (-39.5564, 42.2504) knots 0 0 0 1 1 1
  spline S143 degree 2 poles (-39.5564, 42.2504) (-38.9812, 42.81) (-37.8877, 42.81) knots 0 0 0 1 1 1
  spline S144 degree 2 poles (-37.8877, 42.81) (-36.789, 42.81) (-36.2164, 42.253) knots 0 0 0 1 1 1
  spline S145 degree 2 poles (-36.2164, 42.253) (-35.6439, 41.6959) (-35.6439, 40.6797) knots 0 0 0 1 1 1
  line L119 (-35.6439, 40.6797) -> (-35.6439, 37.2701)
  spline S146 degree 2 poles (-35.6439, 37.2701) (-35.6439, 36.2591) (-36.219, 35.6995) knots 0 0 0 1 1 1
  spline S147 degree 2 poles (-36.219, 35.6995) (-36.7942, 35.1398) (-37.8877, 35.1398) knots 0 0 0 1 1 1
  spline S148 degree 2 poles (-37.8877, 36.5016) (-37.4596, 36.5016) (-37.2584, 36.793) knots 0 0 0 1 1 1
  spline S149 degree 2 poles (-37.2584, 36.793) (-37.0572, 37.0845) (-37.0572, 37.6312) knots 0 0 0 1 1 1
  line L120 (-37.0572, 37.6312) -> (-37.0572, 40.3186)
  spline S150 degree 2 poles (-37.0572, 40.3186) (-37.0572, 40.8654) (-37.2584, 41.1568) knots 0 0 0 1 1 1
  spline S151 degree 2 poles (-37.2584, 41.1568) (-37.4596, 41.4483) (-37.8877, 41.4483) knots 0 0 0 1 1 1
  spline S152 degree 2 poles (-37.8877, 41.4483) (-38.3158, 41.4483) (-38.517, 41.1568) knots 0 0 0 1 1 1
  spline S153 degree 2 poles (-38.517, 41.1568) (-38.7182, 40.8654) (-38.7182, 40.3186) knots 0 0 0 1 1 1
  line L121 (-38.7182, 40.3186) -> (-38.7182, 37.6312)
  spline S154 degree 2 poles (-38.7182, 37.6312) (-38.7182, 37.0845) (-38.517, 36.793) knots 0 0 0 1 1 1
  spline S155 degree 2 poles (-38.517, 36.793) (-38.3158, 36.5016) (-37.8877, 36.5016) knots 0 0 0 1 1 1
  line L122 (-34.4162, 36.4913) -> (-31.8423, 39.875)
  spline S156 degree 2 poles (-31.8423, 39.875) (-31.6669, 40.102) (-31.5715, 40.3418) knots 0 0 0 1 1 1
  spline S157 degree 2 poles (-31.5715, 40.3418) (-31.4761, 40.5817) (-31.4761, 40.788) knots 0 0 0 1 1 1
  line L123 (-31.4761, 40.788) -> (-31.4761, 40.7983)
  spline S158 degree 2 poles (-31.4761, 40.7983) (-31.4761, 41.1027) (-31.6721, 41.2677) knots 0 0 0 1 1 1
  spline S159 degree 2 poles (-31.6721, 41.2677) (-31.8681, 41.4328) (-32.2292, 41.4328) knots 0 0 0 1 1 1
  spline S160 degree 2 poles (-32.2292, 41.4328) (-32.5799, 41.4328) (-32.7966, 41.2033) knots 0 0 0 1 1 1
  spline S161 degree 2 poles (-32.7966, 41.2033) (-33.0132, 40.9737) (-33.0596, 40.5508) knots 0 0 0 1 1 1
  line L124 (-33.0596, 40.5508) -> (-33.0596, 40.5456)
  line L125 (-33.0596, 40.5456) -> (-34.5091, 40.5456)
  line L126 (-34.5091, 40.5456) -> (-34.5091, 40.5508)
  spline S162 degree 2 poles (-34.5091, 40.5508) (-34.4627, 41.2523) (-34.1712, 41.7578) knots 0 0 0 1 1 1
  spline S163 degree 2 poles (-34.1712, 41.7578) (-33.8798, 42.2633) (-33.3846, 42.5289) knots 0 0 0 1 1 1
  spline S164 degree 2 poles (-33.3846, 42.5289) (-32.8894, 42.7946) (-32.2395, 42.7946) knots 0 0 0 1 1 1
  spline S165 degree 2 poles (-32.2395, 42.7946) (-31.538, 42.7946) (-31.0402, 42.565) knots 0 0 0 1 1 1
  spline S166 degree 2 poles (-31.0402, 42.565) (-30.5424, 42.3355) (-30.282, 41.897) knots 0 0 0 1 1 1
  spline S167 degree 2 poles (-30.282, 41.897) (-30.0215, 41.4586) (-30.0215, 40.8396) knots 0 0 0 1 1 1
  line L127 (-30.0215, 40.8396) -> (-30.0215, 40.8345)
  spline S168 degree 2 poles (-30.0215, 40.8345) (-30.0215, 40.3238) (-30.1994, 39.8209) knots 0 0 0 1 1 1
  spline S169 degree 2 poles (-30.1994, 39.8209) (-30.3774, 39.3179) (-30.6972, 38.9105) knots 0 0 0 1 1 1
  line L128 (-30.6972, 38.9105) -> (-32.5438, 36.579)
  line L129 (-32.5438, 36.579) -> (-29.9802, 36.579)
  line L130 (-29.9802, 36.579) -> (-29.9802, 35.2172)
  line L131 (-29.9802, 35.2172) -> (-34.4162, 35.2172)
  line L132 (-34.4162, 35.2172) -> (-34.4162, 36.4913)
  spline S170 degree 2 poles (-26.7512, 35.1398) (-27.4321, 35.1398) (-27.9633, 35.3874) knots 0 0 0 1 1 1
  spline S171 degree 2 poles (-27.9633, 35.3874) (-28.4946, 35.635) (-28.8093, 36.1096) knots 0 0 0 1 1 1
  spline S172 degree 2 poles (-28.8093, 36.1096) (-29.1239, 36.5841) (-29.1549, 37.2392) knots 0 0 0 1 1 1
  line L133 (-29.1549, 37.2392) -> (-27.6951, 37.2392)
  spline S173 degree 2 poles (-27.6951, 37.2392) (-27.6642, 37.0071) (-27.5584, 36.8446) knots 0 0 0 1 1 1
  spline S174 degree 2 poles (-27.5584, 36.8446) (-27.4527, 36.6821) (-27.2876, 36.597) knots 0 0 0 1 1 1
  spline S175 degree 2 poles (-27.2876, 36.597) (-27.1226, 36.5119) (-26.9059, 36.5119) knots 0 0 0 1 1 1
  spline S176 degree 2 poles (-26.9059, 36.5119) (-26.5036, 36.5119) (-26.2844, 36.7363) knots 0 0 0 1 1 1
  spline S177 degree 2 poles (-26.2844, 36.7363) (-26.0651, 36.9607) (-26.0651, 37.3682) knots 0 0 0 1 1 1
  line L134 (-26.0651, 37.3682) -> (-26.0651, 37.5435)
  spline S178 degree 2 poles (-26.0651, 37.5435) (-26.0651, 37.9717) (-26.2431, 38.2038) knots 0 0 0 1 1 1
  spline S179 degree 2 poles (-26.2431, 38.2038) (-26.4211, 38.4359) (-26.7512, 38.4359) knots 0 0 0 1 1 1
  line L135 (-26.7512, 38.4359) -> (-27.3856, 38.4359)
  line L136 (-27.3856, 38.4359) -> (-27.3856, 39.7977)
  line L137 (-27.3856, 39.7977) -> (-26.7512, 39.7977)
  spline S180 degree 2 poles (-26.7512, 39.7977) (-26.4829, 39.7977) (-26.3359, 40.0014) knots 0 0 0 1 1 1
  spline S181 degree 2 poles (-26.3359, 40.0014) (-26.1889, 40.2052) (-26.1889, 40.5714) knots 0 0 0 1 1 1
  line L138 (-26.1889, 40.5714) -> (-26.1889, 40.7003)
  spline S182 degree 2 poles (-26.1889, 40.7003) (-26.1889, 41.0459) (-26.3514, 41.2342) knots 0 0 0 1 1 1
  spline S183 degree 2 poles (-26.3514, 41.2342) (-26.5139, 41.4225) (-26.8079, 41.4225) knots 0 0 0 1 1 1
  spline S184 degree 2 poles (-26.8079, 41.4225) (-26.9988, 41.4225) (-27.1561, 41.3245) knots 0 0 0 1 1 1
  spline S185 degree 2 poles (-27.1561, 41.3245) (-27.3134, 41.2265) (-27.4217, 41.0408) knots 0 0 0 1 1 1
  spline S186 degree 2 poles (-27.4217, 41.0408) (-27.5301, 40.8551) (-27.5765, 40.592) knots 0 0 0 1 1 1
  line L139 (-27.5765, 40.592) -> (-29.0311, 40.592)
  spline S187 degree 2 poles (-29.0311, 40.592) (-28.9692, 41.2781) (-28.6623, 41.7758) knots 0 0 0 1 1 1
  spline S188 degree 2 poles (-28.6623, 41.7758) (-28.3554, 42.2736) (-27.8602, 42.5341) knots 0 0 0 1 1 1
  spline S189 degree 2 poles (-27.8602, 42.5341) (-27.365, 42.7946) (-26.7563, 42.7946) knots 0 0 0 1 1 1
  spline S190 degree 2 poles (-26.7563, 42.7946) (-25.7608, 42.7946) (-25.2166, 42.2865) knots 0 0 0 1 1 1
  spline S191 degree 2 poles (-25.2166, 42.2865) (-24.6724, 41.7784) (-24.6724, 40.8448) knots 0 0 0 1 1 1
  line L140 (-24.6724, 40.8448) -> (-24.6724, 40.6178)
  spline S192 degree 2 poles (-24.6724, 40.6178) (-24.6724, 40.0968) (-24.9355, 39.71) knots 0 0 0 1 1 1
  spline S193 degree 2 poles (-24.9355, 39.71) (-25.1986, 39.3231) (-25.6834, 39.1323) knots 0 0 0 1 1 1
  spline S194 degree 2 poles (-25.6834, 39.1323) (-25.1418, 39.0085) (-24.8452, 38.5649) knots 0 0 0 1 1 1
  spline S195 degree 2 poles (-24.8452, 38.5649) (-24.5486, 38.1212) (-24.5486, 37.4352) knots 0 0 0 1 1 1
  line L141 (-24.5486, 37.4352) -> (-24.5486, 37.2082)
  spline S196 degree 2 poles (-24.5486, 37.2082) (-24.5486, 36.5532) (-24.8065, 36.0889) knots 0 0 0 1 1 1
  spline S197 degree 2 poles (-24.8065, 36.0889) (-25.0645, 35.6247) (-25.5596, 35.3823) knots 0 0 0 1 1 1
  spline S198 degree 2 poles (-25.5596, 35.3823) (-26.0548, 35.1398) (-26.7512, 35.1398) knots 0 0 0 1 1 1
  dimension "d47" = 60
  dimension "d50" = 6.8
  dimension "d51" = 6.8
  dimension "d52" = 6.8
  dimension "d53" = 6.8
  constraint horizontal L23
  constraint vertical L24
  constraint horizontal L25
  constraint vertical L26
  constraint coincident L10 L24.end
  constraint coincident L8.end L9.start
  constraint midpoint L9 L27.start
  constraint midpoint L25 L27.end
  constraint coincident L25 L28.start
  constraint coincident L9 L28.end
  constraint perpendicular L9 L28
  constraint coincident L9 L29.start
  constraint coincident L25 L29.end
  constraint perpendicular L25 L29
  constraint coincident L25 L30.start
  constraint coincident L9 L30.end
  constraint perpendicular L9 L30
  constraint coincident L9 L31.start
  constraint coincident L25 L31.end
  constraint perpendicular L25 L31
  constraint symmetric L27 L28.start L32.start
  constraint symmetric L27 L28.end L32.end
  constraint symmetric L27 L29.start L33.start
  constraint symmetric L27 L29.end L33.end
  constraint symmetric L27 L30.start L34.start
  constraint symmetric L27 L30.end L34.end
  constraint symmetric L27 L31.start L35.start
  constraint symmetric L27 L31.end L35.end
  measures "d47" distance of L23 L25
  measures "d50" distance of L27 L28
  measures "d51" distance of L28 L29
  measures "d52" distance of L29 L30
  measures "d53" distance of L30 L31
extrude "Extrude5" cut sketch "Sketch4" against normal up to surface (2 mm away) contours L33 S91 S92 L84 L85 | L33 S84 S85 S86 S87 L83 S88 S89 S90 S91 L85 L86 L87 L88 L89 L90 S103 | L32 L71 L72 L73 L79 L80 L81 | L32 L71 L74 L79 | L32 S171 S172 L133 | L32 S170 S171 L133 S173 S174 S175 S176 S177 L134 S178 S179 L135 L136 L137 S180 S181 L138 S182 S183 S184 S185 S186 L139 S188 S189 S190 S191 L140 S192 S193 S194 S195 L141 S196 S197 S198 | L32 L79 L80 L81 | L32 L74 L79 L81 | L86 S93 S94 S95 S96 L87 L89 S97 S98 S99 S100 S101 S102 S103 S104 S105 | L86 L90 S103 | L28 S62 L60 | L28 S40 S41 S42 L59 S43 S44 S45 S46 S47 S48 S49 S50 S51 S52 S53 S54 S55 S56 S57 S58 S59 S60 S61 S62 L60 S63 S64 S65 S66 S67 S68 S69 S70 S71 S72 S73 S74 S75 S78 S79 | L32 L73 L74 L81 | L74 L76 L79 L81 | L28 L107 S126 S127 L108 S128 S129 S130 S131 L109 L110 L111 S132 S133 S134 S135 S136 S139 L113 L114 L116 L117 | L28 L114 L115 L116 | L32 L139 S187 S188 | L29 S27 S28 S29 L52 L53 L55 L56 S30 | L29 S21 S22 S23 L51 S24 S25 S26 S27 L53 L54 L55 S30 S31 S32 S33 S34 S35 S36 S37 S39 | L75 L76 L77 L78 L79 L81 L82 | L76 L79 L81 L82 | L29 S37 L58 S38 S39 | L86 L87 L88 L89 | L30 S0 S1 L37 S2 S3 S4 S5 S6 S7 S8 S9 S10 S11 S12 S13 S14 S15 S16 S17 L44 S18 S19 S20 | L30 S8 L41 L43 S9 L48 | L28 S75 S76 S77 S78 | L30 L36 S0 S20 L45 L48 | L28 S136 S137 L112 S138 S139 | L29 L53 L55 S33 L57 S34 | L30 S4 L38 L40 S5 L48 | L41 L42 L43 L47 L48 | L53 L54 L55 S33 L57 S34 | L36 L45 L46 L48 L49 | L36 L38 L39 L40 L41 L42 L46 L47 L48 L49 L50 | L38 L39 L40 L48 | S80 S81 L61 L63 S82 S83 L64 L65 L66 L69 | L61 L67 L69 L70 | L61 L63 L67 L69 | L61 L62 L63 L67 | L63 L67 L68 L69 | S106 S107 S108 L91 S109 S110 S111 S112 S113 S114 L92 S115 S116 S117 S118 L93 S119 S120 S121 S122 L94 S123 S124 S125 | L95 L97 L98 L99 L100 L101 L102 | L95 L97 L98 L100 | L95 L96 L97 L100 L103 L104 L106 | L97 L103 L104 L106 | L97 L104 L105 L106 | S140 S141 L118 S142 S143 S144 S145 L119 S146 S147 | L122 S156 S157 L123 S158 S159 S160 S161 L124 L125 L126 S162 S163 S164 S165 S166 S167 L127 S168 S169 L128 L129 L130 L131 L132